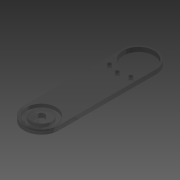
# Autodesk Inventor part: JointC3'B_2nd
Saved by Autodesk Inventor 2011 (Build 150239000, 239)
## iProperties
Created: 2013-02-07
Part Number: JointC3'B_2nd
Document SubType Name: Modeling
Designer: JohnHenry
Density: 1 g/cm^3
Author: JohnHenry
Autodesk Inventor part; units mm, degrees
ref_plane "YZ Plane" through (0, 0, 0) normal (1, 0, 0) x (0, 1, 0)
ref_plane "XZ Plane" through (0, 0, 0) normal (0, 1, 0) x (-1, 0, 0)
ref_plane "XY Plane" through (0, 0, 0) normal (0, 0, 1) x (1, 0, 0)
sketch "スケッチ1" plane through (0, 0, 0) normal (0, 0, 1) x (1, 0, 0)
  line L0 (-15.75, 60) -> (15.75, 60)
  line L1 (15.75, 60) -> (15.75, -60)
  line L2 (15.75, -60) -> (-15.75, -60)
  line L3 (-15.75, -60) -> (-15.75, 60)
  point P0 (0, 0)
  dimension "d0" = 31.5
  dimension "d1" = 15.75
  dimension "d2" = 120
  dimension "d3" = 60
  constraints: 8 end point, 2 parallel, 1 horizontal, 1 perpendicular
  measures "d0" distance of L1.end L2.end
  measures "d1" distance from line of L3 point (0, 0)
  measures "d2" distance of L0.end L1.end
  measures "d3" distance from line of L2 point (0, 0)
extrude "押し出し1" add sketch "スケッチ1" along normal blind 4
fillet "フィレット1" radius 15.75 4 edges at (-15.75, -60, 2) (15.75, -60, 2) (15.75, 60, 2) (-15.75, 60, 2)
sketch "スケッチ2" plane through (0, 0, 4) normal (0, 0, 1) x (1, 0, 0)
  arc A0 (15.75, 44.25) -> (-15.75, 44.25) centre (0, 44.25) ccw projected
  circle A1 centre (0, 44.25) radius 14
  point P0 (0, 0)
  dimension "d7" = 28
  constraints: 1 centre point, 1 coincident
  measures "d7" diameter of A1
extrude "押し出し2" cut sketch "スケッチ2" against normal through all
sketch "スケッチ3" plane through (0, 0, 4) normal (0, 0, 1) x (1, 0, 0)
  arc A0 (15.75, 44.25) -> (-15.75, 44.25) centre (0, 44.25) ccw projected
  circle A1 centre (0, 44.25) radius 19.5
  line L0 (0, 44.25) -> (0, 24.75)
  line L1 (0, 44.25) -> (9.75, 27.3625)
  line L2 (0, 44.25) -> (-9.75, 27.3625)
  line L3 (0, 44.25) -> (0, 63.75)
  point P0 (0, 0)
  point P1 (9.75, 27.3625)
  dimension "d10" = 39
  dimension "d11" = 150
  dimension "d13" = 30
  constraints: 8 end point, 5 point on circle, 3 coincident, 1 centre point, 1 collinear
  measures "d10" diameter of A1
  measures "d11" angle of L1 L3
  measures "d13" angle of L2 L0
hole "Hole1" at (-9.75, 27.3625, 4) at (9.75, 27.3625, 4) at (0, 24.75, 4) direction (0, 0, -1) diameter 3.2 depth 8 tip angle 118
sketch "スケッチ4" plane through (0, 0, 4) normal (0, 0, 1) x (1, 0, 0)
  arc A0 (-15.75, -44.25) -> (15.75, -44.25) centre (0, -44.25) ccw projected
  point P0 (0, 0)
  constraints: 1 coincident
hole "Hole2" at (0, -44.25, 4) direction (0, 0, -1) diameter 6 end through all
sketch "スケッチ5" plane through (0, 0, 4) normal (0, 0, 1) x (1, 0, 0)
  circle A0 centre (0, -44.25) radius 13.25
  circle A1 centre (0, -44.25) radius 9.25
  point P0 (0, 0)
  dimension "d28" = 26.5
  dimension "d29" = 18.5
  constraints: 2 centre point
  measures "d28" diameter of A0
  measures "d29" diameter of A1
extrude "押し出し3" cut sketch "スケッチ5" against normal blind 3
equation "\"d1\" = 0.5 * d0"
equation "\"d3\" = 0.5 * d2"
equation "\"d6\" = 0.5 * d0"
